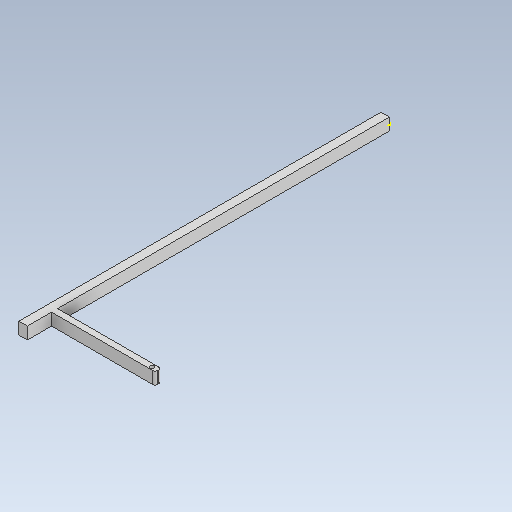
# Autodesk Inventor part: support_rod_left
Saved by Autodesk Inventor 2021 (Build 250183000, 183)
## iProperties
Created: 2021-06-26
Part Number: support_rod_left
Material: Generic
Document SubType Name: Modeling
Designer: TARUN
Density: 1 g/cm^3
Appearance: Default
Author: TARUN
Autodesk Inventor part; units mm, degrees
ref_plane "YZ Plane" through (0, 0, 0) normal (1, 0, 0) x (0, 1, 0)
ref_plane "XZ Plane" through (0, 0, 0) normal (0, 1, 0) x (-1, 0, 0)
ref_plane "XY Plane" through (0, 0, 0) normal (0, 0, 1) x (1, 0, 0)
sketch "Sketch1" plane through (0, 0, 0) normal (0, 0, 1) x (1, 0, 0)
  line L0 (-3.5, -5) -> (3.5, -5)
  line L1 (3.5, -5) -> (3.5, 5)
  line L2 (3.5, 5) -> (-3.5, 5)
  line L3 (-3.5, 5) -> (-3.5, -5)
  line L4 (-3.5, -5) -> (3.5, 5) construction
  line L5 (3.5, -5) -> (-3.5, 5) construction
  point P0 (0, 0)
  dimension "d0" = 7
  dimension "d1" = 10
  constraints: 12 end point, 2 midpoint, 2 parallel, 1 horizontal, 1 perpendicular
  measures "d0" distance of L2.end L1.end
  measures "d1" distance of L1.end L0.end
extrude "Extrusion1" add sketch "Sketch1" along normal blind 300
sketch "Sketch2" plane through (3.5, -5, 0) normal (1, 0, 0) x (0, 0, -1)
  point P0 (0, 5)
sketch "Sketch3" plane through (3.5, -5, 0) normal (1, 0, 0) x (0, 0, -1)
  line L0 (0, 10) -> (-300, 10) projected
  line L1 (0, 0) -> (-300, 0) projected
  line L2 (-275, 10) -> (-280, 10)
  line L3 (-280, 10) -> (-280, 0)
  line L4 (-280, 0) -> (-275, 0)
  line L5 (-275, 0) -> (-275, 10)
  line L6 (-300, 0) -> (-300, 10) projected
  point P0 (0, 5)
  point P1 (-275, 0)
  point P2 (-280, 10)
  dimension "d4" = 5
  dimension "d12" = 20
  constraints: 8 end point, 2 parallel, 2 point on line, 1 horizontal, 1 perpendicular
  measures "d4" distance of L4.end L3.end
  measures "d12" distance between parallel lines of L3 L6
extrude "Extrusion2" add sketch "Sketch3" along normal blind 85.85 contours L5 L1 L3 L0
sketch "Sketch4" plane through (-3.5, 5, 300) normal (0, 1, 0) x (1, 0, 0)
  circle A0 centre (87.8562, 22.5) radius 1.64
  line L0 (7, 25) -> (92.85, 25) projected
  point P0 (3.5, 300)
  dimension "d7" = 3.28
  dimension "d8" = 2.5
  constraints: 1 centre point
  measures "d7" diameter of A0
  measures "d8" distance from line of A0.centre L0
extrude "Extrusion3" cut sketch "Sketch4" against normal through all
fillet "Fillet1" radius 2 2 edges at (89.35, 0, 275) (89.35, 0, 280)
body "Solid1"
